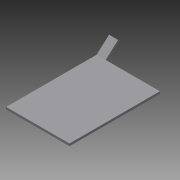
# Autodesk Inventor part: Ball Blocker
Saved by Autodesk Inventor 2014 (Build 180170000, 170)
## iProperties
Created: 2014-01-30
Part Number: Ball Blocker
Material: Generic
Document SubType Name: Modeling
Designer: robotics
Density: 1 g/cm^3
Appearance: Default
Author: robotics
Autodesk Inventor part; units mm, degrees
ref_plane "YZ Plane" through (0, 0, 0) normal (1, 0, 0) x (0, 1, 0)
ref_plane "XZ Plane" through (0, 0, 0) normal (0, 1, 0) x (-1, 0, 0)
ref_plane "XY Plane" through (0, 0, 0) normal (0, 0, 1) x (1, 0, 0)
sketch "Sketch1" plane through (0, 0, 0) normal (1, 0, 0) x (0, 1, 0)
  line L0 (0, 0) -> (6.35, 0)
  line L1 (6.35, 0) -> (6.35, 254)
  line L2 (6.35, 254) -> (0, 254)
  line L3 (0, 254) -> (0, 0)
  line L4 (0, 0) -> (32.6536, -38.9151)
  line L5 (0, 0) -> (50.8, 0) construction
  line L6 (32.6536, -38.9151) -> (37.518, -34.8334)
  line L7 (37.518, -34.8334) -> (6.35, 0)
  dimension "d0" = 6.35
  dimension "d1" = 254
  dimension "d2" = 50.8
  dimension "d3" = 50
  dimension "d4" = 6.35
  constraints: 16 end point, 2 horizontal, 2 parallel, 2 perpendicular, 1 equal length
  measures "d0" distance of L2.end L1.end
  measures "d1" distance of L1.end L0.end
  measures "d2" distance of L0.start L4.end
  measures "d3" angle of L4 L5
  measures "d4" distance of L4.end L6.end
extrude "Extrusion1" add sketch "Sketch1" along normal blind 25.4
sketch "Sketch2" plane through (25.4, 0, 0) normal (1, 0, 0) x (0, 0, -1)
  line L0 (-254, 6.35) -> (-254, 0) projected
  line L1 (-254, 0) -> (0, 0) projected
  line L2 (-254, 6.35) -> (0, 6.35)
  line L3 (0, 6.35) -> (0, 0)
  line L4 (0, 0) -> (-254, 0)
  line L5 (-254, 0) -> (-254, 6.35)
  constraints: 8 end point, 2 parallel, 1 horizontal, 1 perpendicular
extrude "Extrusion2" add sketch "Sketch2" along normal blind 152.4
body "Solid1"
